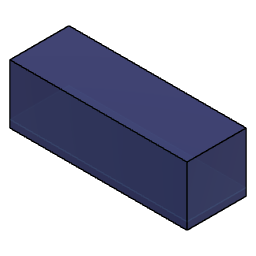
IR Unit (Autodesk Fusion 360 design; units mm, degrees)
Autodesk Fusion 360 part; units mm, degrees
sketch "Sketch2" plane through (0, 0, 0) normal (0, 1, 0) x (1, 0, 0)
  line L0 (20, -30) -> (-40, -30)
  line L1 (-40, -30) -> (-40, -10)
  line L2 (-40, -10) -> (20, -10)
  line L3 (20, -10) -> (20, -30)
  dimension "d7" = 60
  dimension "d8" = 20
  constraint horizontal L0
  constraint perpendicular L0 L1
  constraint parallel L0 L2
  constraint parallel L1 L3
  measures "d7" distance of L1.end L2.end
  measures "d8" distance of L0.start L2.end
extrude "Extrude2" add sketch "Sketch2" along normal blind 2.5
sketch "Sketch3" plane through (0, 2.5, 0) normal (0, 1, 0) x (-1, 0, 0)
  line L0 (-20, 10) -> (40, 10)
  line L1 (40, 10) -> (40, 30)
  line L2 (40, 30) -> (-20, 30)
  line L3 (-20, 30) -> (-20, 10)
sketch "Sketch4" plane through (0, 2.5, 0) normal (0, 1, 0) x (-1, 0, 0)
  line L0 (-18, 28) -> (38, 28)
  line L1 (38, 28) -> (38, 12)
  line L2 (38, 12) -> (-18, 12)
  line L3 (-18, 12) -> (-18, 28)
  line L4 (-18, 28) -> (38, 12) construction
  line L5 (38, 28) -> (-18, 12) construction
  line L6 (-20, 10) -> (40, 10)
  line L7 (40, 30) -> (-20, 30)
  line L8 (-20, 30) -> (-20, 10)
  line L9 (40, 10) -> (40, 30)
  line L10 (30, 8.5) -> (38, 8.5) construction
  point P0 (10, 20)
  dimension "d42" = 2
  dimension "d43" = 2
  dimension "d44" = 2
  dimension "d45" = 2
  constraint horizontal L0
  constraint perpendicular L0 L1
  constraint parallel L0 L2
  constraint parallel L1 L3
  constraint coincident L4 P0
  constraint coincident L5 P0
  constraint coincident L1 L10.end
  constraint perpendicular L1 L10
  measures "d42" distance of L1 L9
  measures "d43" distance of L3 L8
  measures "d44" distance of L2 L6
  measures "d45" distance of L0 L7
sketch "Sketch18" plane through (0, 2.5, 0) normal (0, 1, 0) x (-1, 0, 0)
  line L0 (-20, 10) -> (40, 10)
  line L1 (40, 10) -> (40, 30)
  line L2 (40, 30) -> (-20, 30)
  line L3 (-20, 30) -> (-20, 10)
  line L4 (32.7, -0.7) -> (32.7, 0.8) construction
  line L5 (32.7, 0.8) -> (28.0383, 0.8)
  line L6 (32.7, 0.8) -> (28.0383, 0.8)
  line L7 (32.7, 22.7) -> (32.7, 21.2) construction
  line L8 (32.7, 21.2) -> (28.0383, 21.2)
  line L9 (32.7, 21.2) -> (28.0383, 21.2)
  line L10 (32.7, 22.7) -> (27.8029, 22.7)
  line L11 (32.7, 22.7) -> (37.5971, 22.7)
  line L12 (32.7, -0.7) -> (27.8029, -0.7)
  line L13 (32.7, -0.7) -> (37.5971, -0.7)
  dimension "d140" = 1.5
  dimension "d141" = 1.5
  constraint vertical L4
  constraint perpendicular L4 L5
  constraint perpendicular L4 L6
  constraint perpendicular L6 L7
  constraint perpendicular L7 L8
  constraint perpendicular L7 L9
  constraint perpendicular L7 L10
  constraint perpendicular L7 L11
  constraint perpendicular L4 L12
  constraint perpendicular L4 L13
  measures "d140" distance of L4.start L4.end
  measures "d141" distance of L7.start L7.end
extrude "Extrude7" add sketch "Sketch4" along normal blind 15.5 from surface at -0.5
sketch "Sketch5" plane through (0, 2.5, 0) normal (0, 1, 0) x (-1, 0, 0)
  line L0 (-18, 12) -> (37, 12)
  line L1 (37, 12) -> (37, 19)
  line L2 (37, 19) -> (-18, 19)
  line L3 (-18, 19) -> (-18, 12)
  line L4 (-18, 12) -> (38, 12)
  line L5 (38, 12) -> (38, 20)
  line L6 (38, 20) -> (-18, 20)
  line L7 (-18, 20) -> (-18, 12)
  line L8 (-20, 30) -> (-20, 10)
  line L9 (-20, 10) -> (40, 10)
  dimension "d49" = 55
  dimension "d50" = 7
  dimension "d51" = 1
  dimension "d52" = 1
  dimension "d215" = 2
  dimension "d216" = 2
  constraint horizontal L0
  constraint vertical L1
  constraint horizontal L2
  constraint vertical L3
  constraint horizontal L4
  constraint vertical L5
  constraint horizontal L6
  constraint vertical L7
  measures "d49" distance of L1.end L2.end
  measures "d50" distance of L0.end L1.end
  measures "d51" distance of L2 L6
  measures "d52" distance of L1 L5
  measures "d215" distance of L3 L8
  measures "d216" distance of L4 L9
extrude "Extrude8" add sketch "Sketch5" along normal blind 16 from surface at -0.5 contours L1 L2 L4 L5 L6 L7
sketch "Sketch6" plane through (0, 0, 12) normal (0, 0, 1) x (1, 0, 0)
  line L0 (-37, 2.5) -> (18, 2.5)
  line L1 (18, 2.5) -> (18, 17.5)
  line L2 (18, 17.5) -> (-37, 17.5)
  line L3 (18, 2.5) -> (-37, 2.5)
  line L4 (-37, 2.5) -> (-37, 22)
  line L5 (-37, 22) -> (18, 22)
  line L6 (18, 22) -> (18, 2.5)
  line L7 (16.5, 4) -> (-35.5, 4)
  line L8 (-35.5, 4) -> (-35.5, 16)
  line L9 (-35.5, 16) -> (16.5, 16)
  line L10 (16.5, 16) -> (16.5, 4)
  line L11 (-37, 17.5) -> (-37, 2.5)
  line L12 (-40, 0) -> (20, 0)
  line L13 (16.5, 16) -> (-35.5, 4) construction
  line L14 (-35.5, 16) -> (16.5, 4) construction
  point P0 (-9.5, 10)
  dimension "d57" = 1.5
  dimension "d58" = 1.5
  dimension "d59" = 12
  dimension "d237" = 52
  dimension "d282" = 4
  constraint horizontal L3
  constraint vertical L4
  constraint horizontal L5
  constraint vertical L6
  constraint coincident L0.end L1.start
  constraint horizontal L7
  constraint vertical L8
  constraint horizontal L9
  constraint vertical L10
  constraint midpoint L14 P0
  measures "d57" distance of L6 L10
  measures "d58" distance of L4 L8
  measures "d59" distance of L7 L9
  measures "d237" distance of L8 L10
  measures "d282" distance of L7 L12
extrude "Extrude9" cut sketch "Sketch6" against normal up to surface (2 mm away) contours L7 L8 L9 L10
sketch "Sketch7" plane through (0, 18, 0) normal (0, 1, 0) x (-1, 0, 0)
  line L0 (38, 20) -> (-18, 20)
  line L1 (-18, 19) -> (37, 19)
  line L2 (37, 19) -> (37, 12)
  line L3 (38, 20) -> (-18, 20)
  line L4 (-18, 20) -> (-18, 12)
  line L5 (-18, 12) -> (38, 12)
  line L6 (38, 12) -> (38, 20)
  line L7 (-20, 10) -> (40, 10)
  line L8 (-20, 30) -> (-20, 10)
  line L9 (37, 12) -> (38, 12)
  line L10 (38, 12) -> (38, 20)
  line L11 (-18, 20) -> (-18, 19)
  dimension "d217" = 2
  dimension "d218" = 2
  constraint horizontal L3
  constraint vertical L4
  constraint horizontal L5
  constraint vertical L6
  constraint coincident L0.start L3.start
  measures "d217" distance of L5 L7
  measures "d218" distance of L4 L8
extrude "Extrude11" add sketch "Sketch7" along normal blind 1 from surface at -0.5
sketch "Sketch9" plane through (-38, 0, 0) normal (1, 0, 0) x (0, 0, -1)
  line L0 (-28, 2.5) -> (-20, 2.5)
  line L1 (-20, 17.5) -> (-28, 17.5)
  line L2 (-28, 17.5) -> (-28, 2.5)
  line L3 (-20.5, 6) -> (-28, 6)
  line L4 (-28, 6) -> (-28, 13.5)
  line L5 (-28, 13.5) -> (-20.5, 13.5)
  line L6 (-20.5, 13.5) -> (-20.5, 6)
  line L7 (-20.5, 6) -> (-28, 13.5) construction
  line L8 (-28, 6) -> (-20.5, 13.5) construction
  line L9 (-30, 0) -> (-30, 17.5)
  line L10 (-28, 2.5) -> (-12, 2.5)
  line L11 (-20, 2.5) -> (-20, 17.5)
  line L12 (-30, 0) -> (-10, 0)
  point P0 (-24.25, 9.75)
  dimension "d71" = 5.75
  dimension "d73" = 7.5
  dimension "d74" = 7.5
  dimension "d285" = 3.5
  constraint horizontal L3
  constraint perpendicular L3 L4
  constraint parallel L3 L5
  constraint parallel L4 L6
  constraint coincident L7 P0
  constraint coincident L8 P0
  measures "d71" distance of P0 L9
  measures "d73" distance of L3 L5
  measures "d74" distance of L4.end L5.end
  measures "d285" distance of L3 L10
extrude "Extrude12" cut sketch "Sketch9" against normal up to surface (2 mm away) contours L2 L3 L4 L5 L6
sketch "Sketch14" plane through (0, 0, 19) normal (0, 0, -1) x (-1, 0, 0)
  line L0 (-18, 2.5) -> (37, 2.5)
  line L1 (37, 2.5) -> (37, 17.5)
  line L2 (35.5, 4) -> (-16.5, 4)
  line L3 (-16.5, 4) -> (-16.5, 16)
  line L4 (-18, 17.5) -> (-18, 2.5)
  line L5 (37, 17.5) -> (-18, 17.5)
  line L6 (-16.5, 16) -> (35.5, 4) construction
  line L7 (36.4043, 16.1875) -> (-16.5, 4) construction
  line L8 (-16.5, 16) -> (35.5, 16) construction
  line L9 (36.999, 5.7501) -> (36.999, 14.2501)
  line L10 (32.999, 5.7501) -> (36.999, 14.2501) construction
  line L11 (36.999, 5.7501) -> (32.999, 14.2501) construction
  line L12 (32.999, 14.2501) -> (32.999, 5.7501)
  line L13 (32.999, 5.7501) -> (36.999, 5.7501)
  line L14 (36.999, 14.2501) -> (32.999, 14.2501)
  line L15 (35.5, 16) -> (35.5, 4)
  line L16 (9.5, 10) -> (35.5, 10) construction
  circle A0 centre (-4.001, 10.0001) radius 1.425
  point P0 (9.5, 10)
  point P1 (34.999, 10.0001)
  dimension "d261" = 4
  dimension "d262" = 8.5
  dimension "d264" = 0.0001
  dimension "d274" = 0.001
  dimension "d277" = 2.85
  dimension "d278" = 37
  constraint coincident L3.end L6.start
  constraint coincident L2.start L6.end
  constraint coincident L2.end L3.start
  constraint midpoint L6 P0
  constraint horizontal L13
  constraint perpendicular L9 L13
  constraint parallel L13 L14
  constraint parallel L9 L12
  constraint coincident P0 L16.start
  constraint midpoint L15 L16.end
  constraint midpoint L11 P1
  measures "d261" distance of L9.end L11.end
  measures "d262" distance of L9.end L9.start
  measures "d264" distance of L16 P1
  measures "d274" distance of L1 L9
  measures "d277" diameter of A0
  measures "d278" distance of L12 A0.centre
extrude "Extrude29" cut sketch "Sketch14" against normal up to surface (1 mm away) contours L1 L9 L13 L14 L15 | L12 L13 L14 L15 | A0
sketch "Sketch19" plane through (20, 0, 0) normal (1, 0, 0) x (0, 0, -1)
  line L0 (-30, 17.5) -> (-30, 0)
  line L1 (-30, 0) -> (-10, 0)
  line L2 (-10, 0) -> (-10, 17.5)
  line L3 (-10, 17.5) -> (-30, 17.5)
  point P0 (18, 10)
  point P1 (-27, 10)
sketch "Sketch20" plane through (0, 0, 30) normal (0, 0, 1) x (1, 0, 0)
  line L0 (-40, 17.5) -> (-40, 0)
  line L1 (-40, 0) -> (20, 0)
  line L2 (20, 0) -> (20, 17.5)
  line L3 (20, 17.5) -> (-40, 17.5)
  point P0 (-23.3784, 30.9356)
sketch "Sketch26" plane through (0, 17.5, 0) normal (0, 1, 0) x (-1, 0, 0)
  line L0 (-18, 28) -> (38, 28)
  line L1 (38, 28) -> (38, 20)
  line L2 (40, 10) -> (40, 30)
  line L3 (40, 30) -> (-20, 30)
  line L4 (-20, 30) -> (-20, 10)
  line L5 (-20, 10) -> (40, 10)
  line L6 (40, 10) -> (-20, 10)
  line L7 (-20, 10) -> (-20, 30)
  line L8 (-20, 30) -> (40, 30)
  line L9 (40, 30) -> (40, 10)
  line L10 (38, 12) -> (37, 12)
  line L11 (-18, 19) -> (-18, 20)
  line L12 (-18, 20) -> (-18, 28)
  line L13 (38, 20) -> (38, 12)
  line L14 (37, 12) -> (-18, 12)
  line L15 (-18, 12) -> (-18, 19)
  constraint horizontal L6
  constraint vertical L7
  constraint horizontal L8
  constraint vertical L9
  constraint coincident L3.end L4.start
  constraint coincident L2.start L5.end
extrude "Extrude30" add sketch "Sketch26" along normal blind 2.5 contours L0 L1 L10 L11 L12 L13 L14 L15 | L2 L3 L4 L5 L6 L7 L8 L9
named bodies: "casing body"
